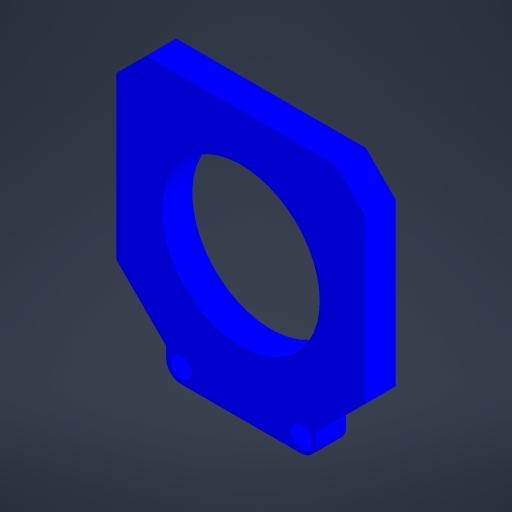
# Autodesk Inventor part: Filter Mount (SM1)
Saved by Autodesk Inventor 2023.4 (Build 274418000, 418)
## iProperties
Created: 2022-11-16
Part Number: Filter Mount (SM1)
Material: Generic
Document SubType Name: Modeling
Designer: xSibe
Density: 1 g/cm^3
Appearance: Plastic Blue
Author: xSibe
Autodesk Inventor part; units mm, degrees
ref_plane "YZ Plane" through (0, 0, 0) normal (1, 0, 0) x (0, 1, 0)
ref_plane "XZ Plane" through (0, 0, 0) normal (0, 1, 0) x (-1, 0, 0)
ref_plane "XY Plane" through (0, 0, 0) normal (0, 0, 1) x (1, 0, 0)
sketch "Sketch1" plane through (0, 0, 0) normal (0, 0, 1) x (1, 0, 0)
  line L0 (139.6, 3.85) -> (159.6, 3.85) construction
  line L1 (139.6, 1.35) -> (159.6, 1.35)
  line L2 (159.6, 6.35) -> (139.6, 6.35)
  arc A0 (139.6, 6.35) -> (139.6, 1.35) centre (139.6, 3.85) ccw
  arc A1 (159.6, 1.35) -> (159.6, 6.35) centre (159.6, 3.85) ccw
  line L3 (137.1, 3.85) -> (162.1, 3.85)
  line L4 (162.1, 3.85) -> (162.1, 7.7)
  line L5 (162.1, 7.7) -> (137.1, 7.7)
  line L6 (137.1, 7.7) -> (137.1, 3.85)
  line L7 (132.55, 42.1) -> (166.65, 42.1)
  line L8 (166.65, 42.1) -> (166.65, 7.7)
  line L9 (166.65, 7.7) -> (132.55, 7.7)
  line L10 (132.55, 7.7) -> (132.55, 42.1)
  line L11 (165.4, 45.85) -> (133.8, 45.85)
  line L12 (128.8, 40.85) -> (128.8, 13.95)
  line L13 (138.8, 3.95) -> (160.4, 3.95)
  line L14 (170.4, 13.95) -> (170.4, 40.85)
  line L15 (128.8, 40.85) -> (133.8, 45.85)
  line L16 (165.4, 45.85) -> (170.4, 40.85)
  line L17 (128.8, 13.95) -> (138.8, 3.95)
  line L18 (160.4, 3.95) -> (170.4, 13.95)
  line L19 (132.55, 24.9) -> (166.65, 24.9)
  circle A2 centre (149.6, 24.9) radius 13.125
  circle A3 centre (139.6, 3.85) radius 1.705
  circle A4 centre (159.6, 3.85) radius 1.705
  line L20 (172.5, 0.025) -> (126.7, 0.025) projected
  line L21 (172.5, 42.1) -> (172.5, 0.025) projected
  line L22 (172.5, 42.1) -> (166.65, 42.1) projected
  line L23 (166.65, 7.7) -> (166.65, 42.1) projected
  line L24 (132.55, 7.7) -> (166.65, 7.7) projected
  line L25 (132.55, 7.7) -> (132.55, 42.1) projected
  line L26 (132.55, 42.1) -> (126.7, 42.1) projected
  line L27 (126.7, 0.025) -> (126.7, 42.1) projected
  circle A5 centre (169.5, 34.8) radius 2.0625 projected
  circle A6 centre (129.7, 34.8) radius 2.0625 projected
  circle A7 centre (169.5, 15) radius 2.0625 projected
  circle A8 centre (129.7, 15) radius 2.0625 projected
  circle A9 centre (159.6, 3.85) radius 1.5625 projected
  circle A10 centre (139.6, 3.85) radius 1.5625 projected
  point P0 (0, 0)
  point P1 (149.6, 3.85)
  point P2 (170.4, 45.85)
  point P3 (128.8, 45.85)
  point P4 (128.8, 3.95)
  point P5 (170.4, 3.95)
  point P6 (137.5172, 5.2328)
  point P7 (161.6828, 5.2328)
  point P8 (162.1, 5.65)
  point P9 (162.1, 3.85)
  point P10 (137.1, 5.65)
  dimension "d0" = 5
  dimension "d1" = 25
  dimension "d2" = 3.75
  dimension "d3" = 5
  dimension "d4" = 5
  dimension "d5" = 5
  dimension "d6" = 5
  dimension "d7" = 10
  dimension "d8" = 10
  dimension "d9" = 10
  dimension "d10" = 10
  dimension "d11" = 26.25
  dimension "d16" = 0.1425
  dimension "d17" = 0.1425
  constraints: 42 end point, 8 point on line, 7 parallel, 6 midpoint, 5 centre point, 5 point on circle, 4 tangent, 3 horizontal, 3 perpendicular, 2 coincident, 3 other
  measures "d0" diameter of A1
  measures "d1" distance of L5.end L4.end
  measures "d2" distance between parallel lines of L7 L11
  measures "d3" distance of L12.start point (128.8, 45.85)
  measures "d4" distance of L11.end point (128.8, 45.85)
  measures "d5" distance of L11.start point (170.4, 45.85)
  measures "d6" distance of L14.end point (170.4, 45.85)
  measures "d7" distance of L12.end point (128.8, 3.95)
  measures "d8" distance of L13.start point (128.8, 3.95)
  measures "d9" distance of L13.end point (170.4, 3.95)
  measures "d10" distance of L14.start point (170.4, 3.95)
  measures "d11" diameter of A2
  measures "d16" radial gap between concentric circles of A3 A10
  measures "d17" radial gap between concentric circles of A4 A9
extrude "Extrusion1" add sketch "Sketch1" along normal mid plane 5 contours A0 L3 A3 A4 A1 L1 | L6 L17 A0 | A0 L17 A3 L3 | L3 A4 L18 A1 | A1 L18 L4 | L17 L6 L5 L4 L18 A1 L2 A0 | A0 L2 A1 L18 A4 L13 A3 L17 | L17 L9 L6 | L4 L9 L18 | A3 L13 A4 L3 | L9 L17 L10 L19 A2 L8 L18 L5 | L17 A8 L12 A6 L15 L26 L10 | L8 L22 L16 L14 A5 A7 L18 | L10 L7 L8 L19 A2 | L17 L12 A8 | A7 L14 L18 | L26 L15 L11 L16 L22 L7 | L12 A6 | A5 L14 picked at (130.3651, 15.6172) picked at (169.0173, 15.7688) picked at (129.7875, 34.8) picked at (169.4174, 34.7184)
equation "\"d4\" = d3"
equation "\"d5\" = d3"
equation "\"d6\" = d5"
equation "\"d8\" = d7"
equation "\"d9\" = d7"
equation "\"d10\" = d9"
body "Solid1"
